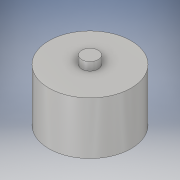
# Autodesk Inventor part: stackLightBase
Saved by Autodesk Inventor 2018 (Build 220112000, 112)
## iProperties
Created: 2017-04-10
Part Number: stackLightBase
Material: ABS Plastic
Document SubType Name: Modeling
Designer: dkt01
Density: 1.06 g/cm^3
Appearance: Aluminum - Polished
Author: dkt01
Autodesk Inventor part; units mm, degrees
ref_plane "YZ Plane" through (0, 0, 0) normal (1, 0, 0) x (0, 1, 0)
ref_plane "XZ Plane" through (0, 0, 0) normal (0, 1, 0) x (-1, 0, 0)
ref_plane "XY Plane" through (0, 0, 0) normal (0, 0, 1) x (1, 0, 0)
sketch "Sketch1" plane through (0, 0, 0) normal (0, 1, 0) x (-1, 0, 0)
  circle A0 centre (0, 0) radius 25
  dimension "d0" = 50
  constraints: 1 centre point, 1 coincident
  measures "d0" diameter of A0
extrude "Extrusion1" add sketch "Sketch1" along normal blind 32
sketch "Sketch2" plane through (0, 32, 0) normal (0, 1, 0) x (1, 0, 0)
  circle A0 centre (0, 0) radius 5
  dimension "d3" = 10
  constraints: 1 centre point, 1 coincident
  measures "d3" diameter of A0
extrude "Extrusion2" add sketch "Sketch2" along normal blind 5
sketch "Sketch3" plane through (0, 0, 0) normal (0, -1, 0) x (1, 0, 0)
  circle A0 centre (0, 0) radius 15
  circle A1 centre (0, 0) radius 5 projected
  circle A2 centre (0, 0) radius 5
  point P0 (15, 0)
  point P1 (-15, 0)
  point P2 (0, -5)
  dimension "d7" = 10
  dimension "d6" = 30
  constraints: 2 coincident, 2 point on circle, 1 centre point, 1 vertical alignment, 2 other
  measures "d6" diameter of A0
hole "Hole1" at (15, 0, 0) at (-15, 0, 0) direction (0, 1, 0) diameter 5 depth 10
hole "Hole2" at (0, 0, -5) direction (0, 1, 0) diameter 8 depth 10
body "Solid1"
